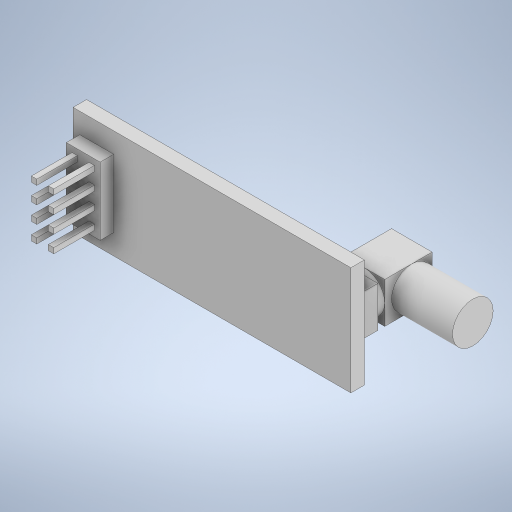
# Autodesk Inventor part: nrf24
Saved by Autodesk Inventor 2024 (Build 280153000, 153)
## iProperties
Created: 2024-03-14
Part Number: nrf24
Material: Générique
Document SubType Name: Modeling
Designer: phaly
Density: 1 g/cm^3
Appearance: Par défaut
Author: phaly
Autodesk Inventor part; units mm, degrees
ref_plane "YZ Plane" through (0, 0, 0) normal (1, 0, 0) x (0, 1, 0)
ref_plane "XZ Plane" through (0, 0, 0) normal (0, 1, 0) x (-1, 0, 0)
ref_plane "XY Plane" through (0, 0, 0) normal (0, 0, 1) x (1, 0, 0)
sketch "Esquisse1" plane through (0, 0, 0) normal (0, 0, 1) x (1, 0, 0)
  line L0 (0, 16) -> (41, 16)
  line L1 (41, 16) -> (41, 0)
  line L2 (41, 0) -> (0, 0)
  line L3 (0, 0) -> (0, 16)
  line L4 (0, -3.2) -> (0, 19.2) projected
  line L5 (-8.2, 0) -> (49.2, 0) projected
  point P0 (0, 0)
  dimension "d0" = 16
  dimension "d1" = 41
  constraints: 8 end point, 2 collinear, 2 parallel, 1 horizontal, 1 perpendicular
  measures "d0" distance of L0.end L1.end
  measures "d1" distance of L0.start L0.end
extrude "Extrusion1" add sketch "Esquisse1" along normal blind 2
sketch "Esquisse2" plane through (0, 0, 2) normal (0, 0, 1) x (1, 0, 0)
  line L0 (1, 13) -> (3.5, 13)
  line L1 (3.5, 13) -> (3.5, 10.5)
  line L2 (3.5, 10.5) -> (1, 10.5)
  line L3 (1, 10.5) -> (1, 13)
  line L4 (3.5, 13) -> (6, 13)
  line L5 (6, 13) -> (6, 10.5)
  line L6 (6, 10.5) -> (3.5, 10.5)
  line L7 (3.5, 10.5) -> (3.5, 13)
  line L8 (0, -3.2) -> (0, 19.2) projected
  line L9 (1, 8) -> (1, 10.5)
  line L10 (1, 10.5) -> (3.5, 10.5)
  line L11 (3.5, 10.5) -> (3.5, 8)
  line L12 (3.5, 10.5) -> (6, 10.5)
  line L13 (6, 10.5) -> (6, 8)
  line L14 (6, 8) -> (3.5, 8)
  line L15 (3.5, 8) -> (1, 8)
  line L16 (1, 5.5) -> (1, 8)
  line L17 (1, 8) -> (3.5, 8)
  line L18 (3.5, 8) -> (3.5, 5.5)
  line L19 (3.5, 8) -> (6, 8)
  line L20 (6, 8) -> (6, 5.5)
  line L21 (6, 5.5) -> (3.5, 5.5)
  line L22 (3.5, 5.5) -> (1, 5.5)
  line L23 (1, 3) -> (1, 5.5)
  line L24 (1, 5.5) -> (3.5, 5.5)
  line L25 (3.5, 5.5) -> (3.5, 3)
  line L26 (3.5, 5.5) -> (6, 5.5)
  line L27 (6, 5.5) -> (6, 3)
  line L28 (6, 3) -> (3.5, 3)
  line L29 (3.5, 3) -> (1, 3)
  line L30 (41, 16) -> (0, 16) projected
  point P0 (0, 0)
  dimension "d4" = 2.5
  dimension "d5" = 2.5
  dimension "d8" = 2.5
  dimension "d9" = 2.5
  dimension "d12" = 2.5
  dimension "d17" = 3
  dimension "d18" = 1
  constraints: 58 end point, 4 parallel, 2 collinear, 2 horizontal, 2 perpendicular, 1 vertical, 45 other
  measures "d4" distance of L0.start L0.end
  measures "d5" distance of L2.end L0.start
  measures "d8" distance of L4.start L4.end
  measures "d9" distance of L4.end L5.end
  measures "d12" distance of L2.end L9.start
  measures "d17" distance between parallel lines of L30 L0
  measures "d18" distance between parallel lines of L8 L3
extrude "Extrusion2" add sketch "Esquisse2" along normal blind 2
sketch "Esquisse3" plane through (0, 0, 4) normal (0, 0, 1) x (1, 0, 0)
  line L0 (1.85, 12.15) -> (2.65, 12.15)
  line L1 (2.65, 12.15) -> (2.65, 11.35)
  line L2 (2.65, 11.35) -> (1.85, 11.35)
  line L3 (1.85, 11.35) -> (1.85, 12.15)
  line L4 (6, 13) -> (1, 13) projected
  line L5 (1, 13) -> (1, 3) projected
  line L6 (2.65, 9.65) -> (2.65, 8.85)
  line L7 (1.85, 9.65) -> (2.65, 9.65)
  line L8 (1.85, 8.85) -> (1.85, 9.65)
  line L9 (2.65, 8.85) -> (1.85, 8.85)
  line L10 (2.65, 7.15) -> (2.65, 6.35)
  line L11 (1.85, 7.15) -> (2.65, 7.15)
  line L12 (1.85, 6.35) -> (1.85, 7.15)
  line L13 (2.65, 6.35) -> (1.85, 6.35)
  line L14 (2.65, 4.65) -> (2.65, 3.85)
  line L15 (1.85, 4.65) -> (2.65, 4.65)
  line L16 (1.85, 3.85) -> (1.85, 4.65)
  line L17 (2.65, 3.85) -> (1.85, 3.85)
  line L18 (5.15, 12.15) -> (5.15, 11.35)
  line L19 (4.35, 12.15) -> (5.15, 12.15)
  line L20 (4.35, 11.35) -> (4.35, 12.15)
  line L21 (5.15, 11.35) -> (4.35, 11.35)
  line L22 (5.15, 9.65) -> (5.15, 8.85)
  line L23 (4.35, 9.65) -> (5.15, 9.65)
  line L24 (4.35, 8.85) -> (4.35, 9.65)
  line L25 (5.15, 8.85) -> (4.35, 8.85)
  line L26 (5.15, 7.15) -> (5.15, 6.35)
  line L27 (4.35, 7.15) -> (5.15, 7.15)
  line L28 (4.35, 6.35) -> (4.35, 7.15)
  line L29 (5.15, 6.35) -> (4.35, 6.35)
  line L30 (5.15, 4.65) -> (5.15, 3.85)
  line L31 (4.35, 4.65) -> (5.15, 4.65)
  line L32 (4.35, 3.85) -> (4.35, 4.65)
  line L33 (5.15, 3.85) -> (4.35, 3.85)
  point P0 (0, 0)
  dimension "d21" = 0.8
  dimension "d22" = 0.8
  dimension "d23" = 0.85
  dimension "d24" = 0.85
  dimension "d27" = 2.5
  dimension "d30" = 2.5
  constraints: 64 end point, 2 horizontal, 2 parallel, 1 perpendicular, 1 vertical, 56 other
  measures "d21" distance of L0.start L0.end
  measures "d22" distance of L2.end L0.start
  measures "d23" distance between parallel lines of L4 L0
  measures "d24" distance between parallel lines of L5 L3
  measures "d27" distance of L0.end L6.start
  measures "d30" distance of L0.end L18.start
extrude "Extrusion3" add sketch "Esquisse3" along normal blind 6
sketch "Esquisse4" plane through (0, 0, 0) normal (0, 0, -1) x (-1, 0, 0)
  line L0 (-40, 5) -> (-34, 5)
  line L1 (-34, 5) -> (-34, 11)
  line L2 (-34, 11) -> (-40, 11)
  line L3 (-40, 11) -> (-40, 5)
  line L4 (-41, 0) -> (-41, 16) projected
  line L5 (0, 0) -> (-41, 0) projected
  dimension "d35" = 6
  dimension "d36" = 6
  dimension "d37" = 1
  dimension "d38" = 5
  constraints: 8 end point, 2 parallel, 1 horizontal, 1 perpendicular
  measures "d35" distance of L2.end L0.start
  measures "d36" distance of L0.start L0.end
  measures "d37" distance between parallel lines of L4 L3
  measures "d38" distance between parallel lines of L5 L0
extrude "Extrusion4" add sketch "Esquisse4" along normal blind 3
sketch "Esquisse5" plane through (0, 0, -3) normal (0, 0, -1) x (-1, 0, 0)
  circle A0 centre (-37, 8) radius 3
  line L0 (-34, 11) -> (-40, 11) projected
  line L1 (-40, 11) -> (-40, 5) projected
  line L2 (-34, 5) -> (-34, 11) projected
  point P0 (0, 0)
  constraints: 3 tangent, 1 centre point
extrude "Extrusion5" add sketch "Esquisse5" along normal blind 1 contours A0
sketch "Esquisse6" plane through (37, 8, -4) normal (0, 0, -1) x (-1, 0, 0)
  line L0 (-3, -3) -> (3, -3)
  line L1 (3, -3) -> (3, 3)
  line L2 (3, 3) -> (-3, 3)
  line L3 (-3, 3) -> (-3, -3)
  line L4 (0, 3) -> (-3, 3) projected
  line L5 (-3, 0) -> (-3, -3) projected
  line L6 (-3, -3) -> (0, -3) projected
  line L7 (3, -3) -> (3, 0) projected
  point P0 (37, -8)
  constraints: 8 end point, 4 collinear, 2 parallel, 1 horizontal, 1 perpendicular
extrude "Extrusion6" add sketch "Esquisse6" along normal blind 7
sketch "Esquisse7" plane through (40, 8, -4) normal (1, 0, 0) x (0, 0, -1)
  circle A0 centre (4, 0) radius 3
  line L0 (7, 3) -> (7, -3) projected
  line L1 (0, -3) -> (7, -3) projected
  line L2 (0, 3) -> (7, 3) projected
  point P0 (-4, -8)
  constraints: 3 tangent, 1 centre point
extrude "Extrusion7" add sketch "Esquisse7" along normal blind 9 contours A0
equation "\"d5\" = d4"
equation "\"d8\" = d4"
equation "\"d9\" = d5"
equation "\"d22\" = d21"
equation "\"d24\" = d23"
equation "\"d36\" = d35"
